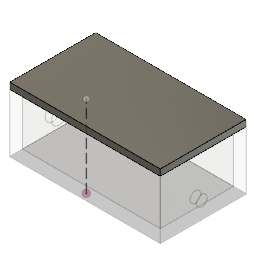
enclosure (Autodesk Fusion 360 design; units mm, degrees)
Autodesk Fusion 360 part; units mm, degrees
sketch "Sketch1" plane through (0, 0, 0) normal (0, 1, 0) x (1, 0, 0) in component "Base"
  line L0 (-32.6179, 5.6203) -> (37.3821, 5.6203)
  line L1 (37.3821, 5.6203) -> (37.3821, -34.3797)
  line L2 (37.3821, -34.3797) -> (-32.6179, -34.3797)
  line L3 (-32.6179, -34.3797) -> (-32.6179, 5.6203)
  dimension "d1" = 70
  dimension "d2" = 40
  measures "d2" distance of origin
extrude "Extrude1" add sketch "Sketch1" along normal blind 27 makes body 1 in component "Base"
sketch "Sketch2" plane through (0, 27, 0) normal (0, 1, 0) x (-1, 0, 0) in component "Base"
  line L0 (32.6179, 34.3797) -> (-37.3821, 34.3797)
  line L1 (-37.3821, 34.3797) -> (-37.3821, -5.6203)
  line L2 (-37.3821, -5.6203) -> (32.6179, -5.6203)
  line L3 (32.6179, -5.6203) -> (32.6179, 34.3797)
  line L4 (29.6179, 31.3797) -> (-34.3821, 31.3797)
  line L5 (-34.3821, 31.3797) -> (-34.3821, -2.6203)
  line L6 (-34.3821, -2.6203) -> (29.6179, -2.6203)
  line L7 (29.6179, -2.6203) -> (29.6179, 31.3797)
  dimension "d5" = 3
extrude "Extrude2" cut sketch "Sketch2" against normal up to surface (24 mm away) contours L4 L5 L6 L7 bodies 1 in component "Base"
sketch "Sketch3" plane through (37.3821, 0, 0) normal (1, 0, 0) x (0, 0, -1) in component "Base"
  line L0 (-34.3797, 0) -> (5.6203, 0)
  line L1 (5.6203, 0) -> (5.6203, 27)
  line L2 (5.6203, 27) -> (-34.3797, 27)
  line L3 (-34.3797, 27) -> (-34.3797, 0)
  circle A0 centre (-15.0561, 7.6221) radius 2.5
  dimension "d8" = 5
  measures "d8" diameter of A0
extrude "Extrude3" cut sketch "Sketch3" against normal blind 5 contours A0 bodies 1 in component "Base"
sketch "Sketch4" plane through (-32.6179, 0, 0) normal (-1, 0, 0) x (0, 0, 1) in component "Base"
  line L0 (-5.6203, 0) -> (34.3797, 0)
  line L1 (34.3797, 0) -> (34.3797, 27)
  line L2 (34.3797, 27) -> (-5.6203, 27)
  line L3 (-5.6203, 27) -> (-5.6203, 0)
  circle A0 centre (14.3797, 7.6221) radius 3.5
  dimension "d11" = 7
  measures "d11" diameter of A0
extrude "Extrude4" cut sketch "Sketch4" against normal blind 10 contours A0 bodies 1 in component "Base"
sketch "Sketch1 (2)" plane through (0, 27, 0) normal (0, 1, 0) x (-1, 0, 0) in component "Lid"
  line L0 (29.6179, -2.6203) -> (-34.3821, -2.6203)
  line L1 (-34.3821, -2.6203) -> (-34.3821, 31.3797)
  line L2 (-34.3821, 31.3797) -> (29.6179, 31.3797)
  line L3 (29.6179, 31.3797) -> (29.6179, -2.6203)
  line L4 (32.6179, 34.3797) -> (-37.3821, 34.3797)
  line L5 (-37.3821, 34.3797) -> (-37.3821, -5.6203)
  line L6 (-37.3821, -5.6203) -> (32.6179, -5.6203)
  line L7 (32.6179, -5.6203) -> (32.6179, 34.3797)
  line L8 (-37.3821, 34.3797) -> (-37.3821, -5.6203)
  line L9 (-37.3821, -5.6203) -> (32.6179, -5.6203)
  line L10 (32.6179, -5.6203) -> (32.6179, 34.3797)
  line L11 (32.6179, 34.3797) -> (-37.3821, 34.3797)
extrude "Extrude1'" add sketch "Sketch1 (2)" along normal blind 3 separate body contours L0 L1 L2 L3 | L4 L5 L6 L7 L8 L9 L10 L11 makes body 2 in component "Lid"
ref_plane "WorkPlane1" through (0, 0, 31.38) normal (0, 0, 1) x (1, 0, 0) in component "Lid"
sketch "Sketch2 (2)" plane through (0, 0, 31.38) normal (0, 0, 1) x (1, 0, 0) in component "Lid"
  line L0 (0, 0) -> (0, 38) construction
ref_plane "WorkPlane2" through (0, 0, 31.38) normal (0, 0, 1) x (1, 0, 0) in component "Lid"
sketch "Sketch3 (2)" plane through (0, 0, 31.38) normal (0, 0, 1) x (1, 0, 0) in component "Lid"
  line L0 (-32.6179, 27) -> (37.3821, 27)
  line L1 (26, 27) -> (26, 24)
  line L2 (26, 24) -> (-26, 24)
  line L3 (-26, 24) -> (-26, 27)
  line L4 (0, 0) -> (0, 38)
  dimension "d20" = 3
extrude "Extrude2'" add sketch "Sketch3 (2)" against normal blind 1.6 bodies 2 in component "Lid"
ref_plane "WorkPlane3" through (0, 0, -2.62) normal (0, 0, 1) x (1, 0, 0) in component "Lid"
sketch "Sketch4 (2)" plane through (0, 0, -2.62) normal (0, 0, 1) x (1, 0, 0) in component "Lid"
  line L0 (-32.6179, 27) -> (37.3821, 27)
  line L1 (26, 27) -> (26, 24)
  line L2 (26, 24) -> (-26, 24)
  line L3 (-26, 24) -> (-26, 27)
extrude "Extrude3'" add sketch "Sketch4 (2)" along normal blind 1.6 bodies 2 in component "Lid"
ref_plane "WorkPlane4" through (-29.618, 0, 0) normal (1, 0, 0) x (0, 1, 0) in component "Lid"
sketch "Sketch5" plane through (-29.618, 0, 0) normal (1, 0, 0) x (0, 0, -1) in component "Lid"
  line L0 (-34.3797, 27) -> (5.6203, 27)
  line L1 (-0.0952, 27) -> (-0.0952, 24)
  line L2 (-0.0952, 24) -> (-27, 24)
  line L3 (-27, 24) -> (-27, 27)
extrude "Extrude4'" add sketch "Sketch5" along normal blind 1.6 bodies 2 in component "Lid"
ref_plane "WorkPlane5" through (34.382, 0, 0) normal (1, 0, 0) x (0, 1, 0) in component "Lid"
sketch "Sketch6" plane through (34.382, 0, 0) normal (1, 0, 0) x (0, 0, -1) in component "Lid"
  line L0 (5.6203, 27) -> (-34.3797, 27)
  line L1 (-0.0952, 27) -> (-0.0952, 24)
  line L2 (-0.0952, 24) -> (-27, 24)
  line L3 (-27, 24) -> (-27, 27)
extrude "Extrude5" add sketch "Sketch6" against normal blind 1.6 bodies 2 in component "Lid"
component "Base" placed x (1, 0, 0) y (0, 1, 0) z (0, 0, 1) at (0, 0, 0)
component "Lid" placed x (1, 0, 0) y (0, 1, 0) z (0, 0, 1) at (0, 0, 0)
